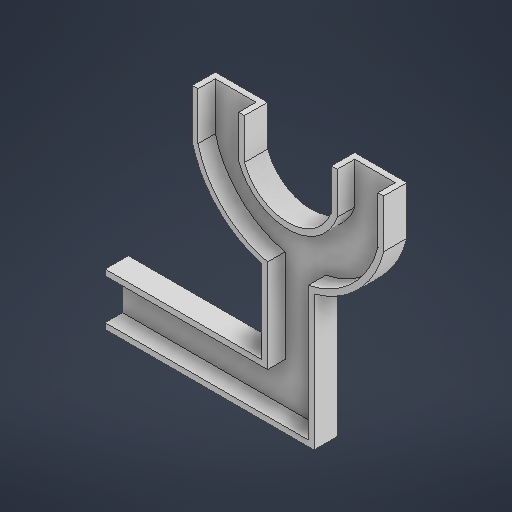
# Autodesk Inventor part: storrageout
Saved by Autodesk Inventor 2026.2 (Build 302298000, 298)
## iProperties
Created: 2026-04-16
Part Number: storrageout
Material: Generic
Document SubType Name: Modeling
Designer: danda
Density: 1 g/cm^3
Appearance: Default
Author: danda
Autodesk Inventor part; units mm, degrees
ref_plane "YZ Plane" through (0, 0, 0) normal (1, 0, 0) x (0, 1, 0)
ref_plane "XZ Plane" through (0, 0, 0) normal (0, 1, 0) x (-1, 0, 0)
ref_plane "XY Plane" through (0, 0, 0) normal (0, 0, 1) x (1, 0, 0)
sketch "Sketch1" plane through (0, 0, 0) normal (0, 0, 1) x (1, 0, 0)
  arc A0 (-37.5, -13.9194) -> (37.5, -13.9194) centre (0, 0) ccw
  line L0 (-37.5, -13.9194) -> (-37.5, 21.0806)
  line L1 (37.5, -13.9194) -> (37.5, 21.0806)
  arc A1 (-42.5, -14.7902) -> (42.5, -14.7902) centre (0, 0) ccw
  line L2 (-42.5, -14.7902) -> (-42.5, 21.0806)
  line L3 (42.5, -14.7902) -> (42.5, 21.0806)
  line L4 (77.5, 21.0806) -> (77.5, -19.8431)
  line L5 (-77.5, -19.8431) -> (-77.5, 21.0806)
  line L6 (82.5, 21.0806) -> (82.5, -20.4634)
  line L7 (-82.5, -20.4634) -> (-82.5, 21.0806)
  line L8 (17.5, -118.4107) -> (17.5, -78.0625)
  line L9 (-17.5, -118.4107) -> (-17.5, -78.0625)
  line L10 (22.5, -81.968) -> (22.5, -123.4107)
  line L11 (-22.5, -123.4107) -> (-22.5, -81.968)
  line L12 (22.5, -123.4107) -> (17.5, -123.4107)
  line L13 (-17.5, -123.4107) -> (-22.5, -123.4107)
  arc A2 (-77.5, -19.8431) -> (-17.5, -78.0625) centre (0, 0) ccw
  arc A3 (17.5, -78.0625) -> (77.5, -19.8431) centre (0, 0) ccw
  arc A4 (-82.5, -20.4634) -> (-22.5, -81.968) centre (0, 0) ccw
  arc A5 (22.5, -81.968) -> (82.5, -20.4634) centre (0, 0) ccw
  line L14 (-17.5, -118.4107) -> (-17.5, -123.4107)
  line L15 (17.5, -118.4107) -> (17.5, -123.4107)
  line L16 (-82.5, 21.0806) -> (-77.5, 21.0806)
  line L17 (-42.5, 21.0806) -> (-37.5, 21.0806)
  line L18 (37.5, 21.0806) -> (42.5, 21.0806)
  line L19 (77.5, 21.0806) -> (82.5, 21.0806)
  line L20 (-22.5, -13.9194) -> (-17.5, -13.9194)
  line L21 (17.5, -13.9194) -> (22.5, -13.9194)
  line L22 (-77.5, 21.0806) -> (82.5, 21.0806)
  line L23 (-17.5, -123.4107) -> (17.5, -123.4107)
  line L24 (22.5, -123.4107) -> (22.5, -163.4107)
  line L25 (22.5, -163.4107) -> (17.5, -163.4107)
  line L26 (17.5, -163.4107) -> (17.5, -123.4107)
  line L27 (-17.5, -123.4107) -> (-17.5, -158.4107)
  line L28 (-22.5, -158.4107) -> (-22.5, -123.4107)
  line L29 (22.5, -163.4107) -> (22.5, -198.4107)
  line L30 (22.5, -198.4107) -> (-157.5, -198.4107)
  line L31 (17.5, -163.4107) -> (17.5, -193.4107)
  line L32 (17.5, -193.4107) -> (-157.5, -193.4107)
  line L33 (-17.5, -158.4107) -> (-157.5, -158.4107)
  line L34 (-157.5, -153.4107) -> (-22.5, -153.4107)
  line L35 (-22.5, -153.4107) -> (-22.5, -123.4107)
  line L36 (-157.5, -198.4107) -> (-157.5, -153.4107)
  point P0 (-22.5, -153.4107)
  dimension "d0" = 75
  dimension "d1" = 40
  dimension "d2" = 35
  dimension "d3" = 35
  dimension "d4" = 5
  dimension "d5" = 5
  dimension "d6" = 5
  dimension "d9" = 35
  dimension "d10" = 20
  dimension "d11" = 5
  dimension "d12" = 0
  dimension "d13" = 0
  dimension "d14" = 5
  dimension "d21" = 35
  dimension "d22" = 180
  dimension "d23" = 175
  dimension "d24" = 5
  dimension "d26" = 144.4913
  dimension "d27" = 40
  dimension "d29" = 5
  constraints: 74 end point, 12 point on circle, 9 point on line, 8 horizontal, 7 parallel, 7 vertical, 6 centre point, 3 perpendicular
  measures "d0" distance of L0.start L1.start
  measures "d1" radius of A0
  measures "d2" distance of L0.start L0.end
  measures "d3" distance of L1.start L1.end
  measures "d4" radial gap between concentric circles of A0 A1
  measures "d5" distance between parallel lines of L0 L2
  measures "d6" distance between parallel lines of L1 L3
  measures "d9" distance of L9.start L8.start
  measures "d10" horizontal distance of L1.start L8.start
  measures "d11" distance between parallel lines of L7 L5
  measures "d12" distance of point (0, 0) A0.centre
  measures "d13" distance of point (0, 0) A0.centre
  measures "d14" distance between parallel lines of L8 L10
  measures "d21" distance of L24.end L29.end
  measures "d22" distance of L29.end L30.end
  measures "d23" distance of L31.end L32.end
  measures "d24" distance between parallel lines of L30 L32
  measures "d26" distance between parallel lines of L23 L22
  measures "d27" distance between parallel lines of L25 L23
  measures "d29" distance between parallel lines of L33 L34
extrude "Extrusion1" add sketch "Sketch1" along normal blind 20 contours A0 L1 L18 L3 A1 L2 L17 L0 | L5 A2 L9 L14 L13 L11 A4 L7 L16 | L19 L6 A5 L10 L12 L15 L8 A3 L4 | L27 L33 L28 L13 | L12 L24 L25 L26 | L28 L33 L36 L34 | L25 L29 L30 L36 L32 L31
extrude "Extrusion2" add sketch "Sketch1" along normal blind 5 contours L2 A1 L3 L22 L4 A3 L8 L15 L23 L14 L9 A2 L5 | L23 L26 L31 L32 L36 L33 L27
equation "\"d3\" = d2"
body "Solid1"
